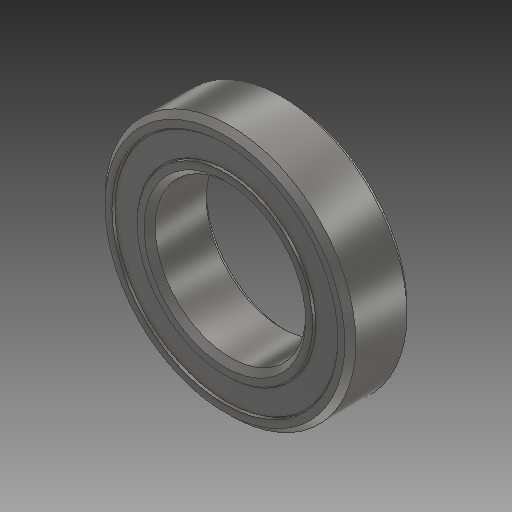
# Autodesk Inventor part: R1038_ZZ_W Bearing
Saved by Autodesk Inventor 2018.2 (Build 222227000, 227)
## iProperties
Created: 2018-02-12
Part Number: R1038_ZZ_W Bearing
Material: Stainless Steel
Document SubType Name: Modeling
Designer: Moochster
Density: 8 g/cm^3
Appearance: Semi-Polished
Mass: 3.79352 g
Surface Area: 5.90649 cm^2
Volume: 0.474189 cm^3
Author: Moochster
Autodesk Inventor part; units mm, degrees
ref_plane "YZ Plane" through (0, 0, 0) normal (1, 0, 0) x (0, 1, 0)
ref_plane "XZ Plane" through (0, 0, 0) normal (0, 1, 0) x (-1, 0, 0)
ref_plane "XY Plane" through (0, 0, 0) normal (0, 0, 1) x (1, 0, 0)
sketch "Sketch1" plane through (0, 0, 0) normal (0, 0, 1) x (1, 0, 0)
  line L0 (0, 0) -> (0, 3.1469)
  line L1 (4.7625, 0) -> (4.7625, 3.937)
  line L2 (4.7625, 3.937) -> (5.55, 3.937)
  line L3 (5.55, 3.937) -> (5.55, 3.737)
  line L4 (5.55, 3.737) -> (5.65, 3.737)
  line L5 (5.65, 3.737) -> (5.65, 3.837)
  line L6 (5.65, 3.837) -> (7.05, 3.837)
  line L7 (7.05, 3.837) -> (7.05, 3.737)
  line L8 (7.05, 3.737) -> (7.15, 3.737)
  line L9 (7.15, 3.737) -> (7.15, 3.937)
  line L10 (7.15, 3.937) -> (7.9375, 3.937)
  line L11 (7.9375, 3.937) -> (7.9375, 0)
  line L12 (7.9375, 0) -> (7.15, 0)
  line L13 (7.15, 0) -> (7.15, 0.25)
  line L14 (7.15, 0.25) -> (7.05, 0.25)
  line L15 (7.05, 0.25) -> (7.05, 0.1)
  line L16 (7.05, 0.1) -> (5.65, 0.1)
  line L17 (5.65, 0.1) -> (5.65, 0.25)
  line L18 (5.65, 0.25) -> (5.55, 0.25)
  line L19 (5.55, 0.25) -> (5.55, 0)
  line L20 (5.55, 0) -> (4.7625, 0)
  line L21 (4.7625, 1.9685) -> (7.9375, 1.9685) construction
  point P0 (6.35, 0.1)
  point P1 (6.35, 1.9685)
  dimension "d0" = 9.525
  dimension "d1" = 3.937
  dimension "d2" = 15.875
  dimension "d3" = 0.1
  dimension "d4" = 0.25
  dimension "d5" = 0.1
  dimension "d6" = 0.1
  dimension "d7" = 1.4
  dimension "d8" = 0.2
  constraints: 44 end point, 15 perpendicular, 7 point on line, 4 horizontal alignment, 4 midpoint, 3 vertical, 3 vertical alignment, 1 other
  measures "d0" diameter of L1 L0
  measures "d1" distance of L1.start L1.end
  measures "d2" diameter of L11 L0
  measures "d3" distance between parallel lines of L20 L16
  measures "d4" distance between parallel lines of L20 L14
  measures "d5" distance of L17.end L18.end
  measures "d6" distance of L13.end L14.end
  measures "d7" distance of L15.end L16.end
  measures "d8" distance between parallel lines of L2 L4
revolve "Revolution1" add sketch "Sketch1" angle 360 about axis through (0, 0, 0) along (0, 1, 0)
chamfer "Chamfer1" distance 0.35 angle 45 4 edges at (-4.7625, 3.937, 0) (-7.9375, 3.937, 0) (-7.9375, 0, 0) (-4.7625, 0, 0)
body "Solid1"
